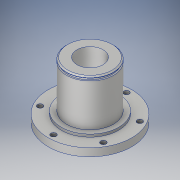
# Autodesk Inventor part: FLY_006_HoodPivot
Saved by Autodesk Inventor 2018.3 (Build 223284000, 284)
## iProperties
Created: 2020-02-09
Part Number: FLY_006_HoodPivot
Material: Aluminum 6061
Document SubType Name: Modeling
Designer: myerpaul
Density: 2.7 g/cm^3
Appearance: Aluminum - Flat
Author: myerpaul
Autodesk Inventor part; units mm, degrees
ref_plane "YZ Plane" through (0, 0, 0) normal (1, 0, 0) x (0, 1, 0)
ref_plane "XZ Plane" through (0, 0, 0) normal (0, 1, 0) x (-1, 0, 0)
ref_plane "XY Plane" through (0, 0, 0) normal (0, 0, 1) x (1, 0, 0)
sketch "Sketch1" plane through (0, 0, 0) normal (0, 0, 1) x (1, 0, 0)
  line L0 (0, 0) -> (0, 30.8582)
  line L1 (7.9375, 1.905) -> (7.9375, 34.544)
  line L2 (7.9375, 34.544) -> (14.2875, 34.544)
  line L3 (14.2875, 34.544) -> (14.2875, 6.35)
  line L4 (17.4625, 4.7625) -> (25.4, 4.7625)
  line L5 (25.4, 4.7625) -> (25.4, 0)
  line L6 (25.4, 0) -> (15.875, 0)
  line L7 (7.9375, 1.905) -> (15.875, 1.905)
  line L8 (15.875, 1.905) -> (15.875, 0)
  line L9 (14.2875, 6.35) -> (17.4625, 6.35)
  line L10 (17.4625, 6.35) -> (17.4625, 4.7625)
  dimension "d0" = 50.8
  dimension "d1" = 15.875
  dimension "d2" = 28.575
  dimension "d3" = 4.7625
  dimension "d19" = 31.75
  dimension "d20" = 1.905
  dimension "d30" = 34.925
  dimension "d31" = 1.5875
  dimension "d34" = 34.544
  constraints: 22 end point, 7 perpendicular, 2 horizontal, 2 vertical, 1 point on line
  measures "d0" diameter of L5 L0
  measures "d1" diameter of L1 L0
  measures "d2" diameter of L3 L0
  measures "d3" distance between parallel lines of L4 L6
  measures "d19" diameter of L8 L0
  measures "d20" distance between parallel lines of L6 L7
  measures "d30" diameter of L10 L0
  measures "d31" distance of L9.end L4.start
  measures "d34" distance between parallel lines of L6 L2
revolve "Revolution1" add sketch "Sketch1" angle 360 about axis through (0, 0, 0) along (0, 1, 0)
sketch "Sketch4" plane through (0, 0, 0) normal (0, 0, 1) x (1, 0, 0)
  line L0 (13.4493, 33.6296) -> (17.9779, 33.6296)
  line L1 (17.9779, 33.6296) -> (17.9779, 32.131)
  line L2 (17.9779, 32.131) -> (13.4493, 32.131)
  line L3 (13.4493, 32.131) -> (13.4493, 33.6296)
  line L4 (-25.4, 4.7625) -> (25.4, 4.7625) projected
  line L5 (-14.2875, 34.544) -> (14.2875, 34.544) projected
  line L6 (0, 34.544) -> (0, 40.6447)
  line L7 (-17.4625, 6.35) -> (17.4625, 6.35) projected
  point P0 (0, 0)
  dimension "d26" = 1.4986
  dimension "d27" = 26.8986
  dimension "d33" = 25.781
  constraints: 10 end point, 2 parallel, 1 horizontal, 1 midpoint, 1 perpendicular, 1 vertical
  measures "d26" distance of L0.end L1.end
  measures "d27" diameter of L3 L6
  measures "d33" distance between parallel lines of L2 L7
revolve "Revolution2" cut sketch "Sketch4" angle 360 about axis through (0, 34.544, 0) along (0, 1, 0)
chamfer "Chamfer1" distance 0.762 angle 45 1 edges at (-14.2875, 34.544, 0)
sketch "Sketch2" plane through (0, 0, 0) normal (0, -1, 0) x (1, 0, 0)
  circle A0 centre (0, 0) radius 22.225 construction
  point P0 (0, -22.225)
  point P1 (19.2474, -11.1125)
  point P2 (19.2474, 11.1125)
  point P3 (0, 22.225)
  point P4 (-19.2474, 11.1125)
  point P5 (-19.2474, -11.1125)
  dimension "d7" = 44.45
  dimension "d10" = 360
  constraints: 2 vertical alignment, 1 coincident, 9 other
hole "Hole1" at (0, 0, -22.225) at (19.2474, 0, -11.1125) at (19.2474, 0, 11.1125) at (0, 0, 22.225) at (-19.2474, 0, 11.1125) at (-19.2474, 0, -11.1125) direction (0, 1, 0) diameter 3.302 end through all thread size "8-32 UNC" class "2B" standard "ANSI Unified Screw Threads"
body "Solid1"
